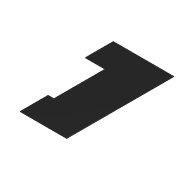
# Autodesk Inventor part: Board_V1
Saved by Autodesk Inventor 2012 (Build 160160000, 160)
## iProperties
Created: 2012-01-21
Part Number: Board_V1
Material: ABS Plastic
Document SubType Name: Modeling
Designer: JesseK
Density: 1.06 g/cm^3
Mass: 508.624 g
Surface Area: 3082.66 cm^2
Volume: 479.834 cm^3
Author: JesseK
Autodesk Inventor part; units mm, degrees
ref_plane "YZ Plane" through (0, 0, 0) normal (1, 0, 0) x (0, 1, 0)
ref_plane "XZ Plane" through (0, 0, 0) normal (0, 1, 0) x (-1, 0, 0)
ref_plane "XY Plane" through (0, 0, 0) normal (0, 0, 1) x (1, 0, 0)
sketch "Sketch1" plane through (0, 0, 0) normal (0, 0, 1) x (1, 0, 0)
  line L0 (0, 0) -> (254, 0)
  line L1 (254, 0) -> (254, 3.175)
  line L2 (254, 3.175) -> (0, 3.175)
  line L3 (0, 3.175) -> (0, 0)
  dimension "d0" = 254
  dimension "d1" = 3.175
  constraints: 8 end point, 2 parallel, 1 coincident, 1 horizontal, 1 perpendicular
  measures "d0" distance of L0.start L0.end
  measures "d1" distance of L2.end L0.start
extrude "Extrusion1" add sketch "Sketch1" along normal blind 584.2
sketch "Sketch2" plane through (0, 3.175, 0) normal (0, 1, 0) x (1, 0, 0)
  line L0 (0, -584.2) -> (254, -584.2) projected
  line L1 (254, 0) -> (0, 0) projected
  line L2 (0, 0) -> (0, -584.2) projected
  line L3 (0, -152.4) -> (31.75, -152.4)
  line L4 (31.75, -152.4) -> (31.75, -431.8)
  line L5 (31.75, -431.8) -> (0, -431.8)
  line L6 (0, -431.8) -> (0, -152.4)
  line L7 (31.75, -152.4) -> (31.75, 0) construction
  line L8 (31.75, -431.8) -> (31.75, -584.2) construction
  dimension "d4" = 31.75
  dimension "d5" = 279.4
  constraints: 12 end point, 3 point on line, 2 parallel, 2 vertical, 1 collinear, 1 horizontal, 1 perpendicular
  measures "d4" distance of L3.start L3.end
  measures "d5" distance of L3.end L4.end
extrude "Extrusion2" cut sketch "Sketch2" against normal through all
sketch "Sketch3" plane through (0, 0, 0) normal (-1, 0, 0) x (0, 0, 1)
  line L0 (0, 0) -> (152.4, 0)
  line L1 (152.4, 0) -> (152.4, 3.175)
  line L2 (152.4, 3.175) -> (0, 3.175)
  line L3 (0, 3.175) -> (0, 0)
  constraints: 8 end point, 2 parallel, 1 horizontal, 1 perpendicular
extrude "Extrusion3" add sketch "Sketch3" along normal blind 76.2
body "Solid1"
